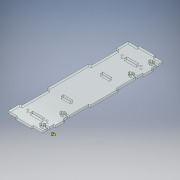
# Autodesk Inventor part: Cubierta_Ducto_Motor
Saved by Autodesk Inventor 2019 (Build 230136000, 136)
## iProperties
Created: 2020-04-03
Part Number: Cubierta_Ducto_Motor
Material: Generic
Document SubType Name: Modeling
Designer: Jurgen
Density: 1 g/cm^3
Appearance: Clear
Mass: 92.9987 g
Surface Area: 415.008 cm^2
Volume: 92.9987 cm^3
Author: Jurgen
Autodesk Inventor part; units mm, degrees
ref_plane "YZ Plane" through (0, 0, 0) normal (1, 0, 0) x (0, 1, 0)
ref_plane "XZ Plane" through (0, 0, 0) normal (0, 1, 0) x (-1, 0, 0)
ref_plane "XY Plane" through (0, 0, 0) normal (0, 0, 1) x (1, 0, 0)
sketch "Sketch1" plane through (0, 0, 0) normal (0, 1, 0) x (-1, 0, 0)
  line L0 (-25, -150) -> (25, -150)
  line L1 (25, 150) -> (-25, 150)
  line L2 (-25, 150) -> (-25, -150)
  line L3 (-25, -150) -> (25, 150) construction
  line L4 (25, -150) -> (-25, 150) construction
  line L5 (25, 150) -> (50, 150)
  line L6 (50, 150) -> (50, 105)
  line L7 (50, 105) -> (45, 105)
  line L8 (25, -150) -> (50, -150)
  line L9 (50, -150) -> (50, -105)
  line L10 (50, -105) -> (45, -105)
  line L11 (50, 105) -> (45, 105) construction
  line L12 (45, 105) -> (45, 45) construction
  line L13 (45, 45) -> (50, 45) construction
  line L14 (50, 45) -> (50, 105) construction
  line L15 (50, -105) -> (45, -105) construction
  line L16 (45, -105) -> (45, -45) construction
  line L17 (45, -45) -> (50, -45) construction
  line L18 (50, -45) -> (50, -105) construction
  line L19 (45, 45) -> (50, 45)
  line L20 (50, 45) -> (50, -45)
  line L21 (50, -45) -> (45, -45)
  line L22 (45, 105) -> (45, 45)
  line L23 (45, -45) -> (45, -105)
  point P0 (0, 0)
  dimension "d1" = 300
  dimension "d8" = 5
  dimension "d10" = 5
  dimension "d11" = 45
  dimension "d13" = 60
  dimension "d14" = 75
  dimension "d15" = 75
  dimension "d29" = 90
  dimension "d30" = 45
  dimension "d31" = 60
  constraints: 48 end point, 8 parallel, 6 horizontal, 5 perpendicular, 2 midpoint, 2 vertical
  measures "d1" distance of L1.start L0.end
  measures "d8" distance of L7.end L6.end
  measures "d10" distance of L10.end L9.end
  measures "d11" distance of L9.end L8.end
  measures "d13" distance of L16.end L15.end
  measures "d14" distance between parallel lines of L2 L9
  measures "d15" distance between parallel lines of L2 L6
  measures "d29" distance of L19.end L17.end
  measures "d30" distance of L5.end L6.end
  measures "d31" distance of L11.end L12.end
extrude "Extrusion1" add sketch "Sketch1" along normal blind 5
sketch "Sketch2" plane through (0, 5, 0) normal (0, 1, 0) x (1, 0, 0)
  line L0 (25, 150) -> (-50, 150) construction
  line L1 (-50, 150) -> (-50, 105) construction
  line L2 (-50, 105) -> (-45, 105) construction
  line L3 (-45, 105) -> (-45, 45) construction
  line L4 (-45, 45) -> (-50, 45) construction
  line L5 (-50, 45) -> (-50, -45) construction
  line L6 (-50, -45) -> (-45, -45) construction
  line L7 (-45, -45) -> (-45, -105) construction
  line L8 (-45, -105) -> (-50, -105) construction
  line L9 (-50, -105) -> (-50, -150) construction
  line L10 (-50, -150) -> (25, -150) construction
  line L11 (25, -150) -> (25, 150) construction
  line L12 (-50, -150) -> (25, -150)
  line L13 (25, -150) -> (25, -130)
  line L14 (25, -130) -> (-50, -130)
  line L15 (-50, -130) -> (-50, -150)
  line L16 (25, -150) -> (25, 150) projected
  line L17 (-50, 150) -> (25, 150)
  line L18 (25, 150) -> (25, 130)
  line L19 (25, 130) -> (-50, 130)
  line L20 (-50, 130) -> (-50, 150)
  point P0 (0, 0)
  dimension "d16" = 20
  dimension "d17" = 20
  constraints: 16 end point, 4 parallel, 2 horizontal, 2 perpendicular, 2 point on line
  measures "d16" distance of L13.end L12.end
  measures "d17" distance of L17.end L18.end
extrude "Extrusion2" cut sketch "Sketch2" against normal blind 5
sketch "Sketch3" plane through (0, 5, 0) normal (0, 1, 0) x (1, 0, 0)
  line L0 (-50, -130) -> (25, -130) construction
  line L1 (25, -130) -> (25, 130) construction
  line L2 (25, 130) -> (-50, 130) construction
  line L3 (-50, 130) -> (-50, 105) construction
  line L4 (-50, 105) -> (-45, 105) construction
  line L5 (-45, 105) -> (-45, 45) construction
  line L6 (-45, 45) -> (-50, 45) construction
  line L7 (-50, 45) -> (-50, -45) construction
  line L8 (-50, -45) -> (-45, -45) construction
  line L9 (-45, -45) -> (-45, -105) construction
  line L10 (-45, -105) -> (-50, -105) construction
  line L11 (-50, -105) -> (-50, -130) construction
  line L12 (2.5, 100) -> (-22.5, 100)
  line L13 (-22.5, 100) -> (-22.5, 95)
  line L14 (-22.5, 95) -> (2.5, 95)
  line L15 (2.5, 95) -> (2.5, 100)
  line L16 (2.5, -109) -> (-22.5, -109)
  line L17 (-22.5, -109) -> (-22.5, -104)
  line L18 (-22.5, -104) -> (2.5, -104)
  line L19 (2.5, -104) -> (2.5, -109)
  point P0 (0, 0)
  dimension "d20" = 25
  dimension "d21" = 5
  dimension "d22" = 22.5
  dimension "d23" = 35
  dimension "d26" = 5
  dimension "d27" = 25
  dimension "d28" = 26
  dimension "d32" = 22.5
  constraints: 16 end point, 2 parallel, 1 horizontal, 1 perpendicular
  measures "d20" distance of L14.end L13.end
  measures "d21" distance of L13.end L12.end
  measures "d22" distance between parallel lines of L1 L15
  measures "d23" distance between parallel lines of L2 L14
  measures "d26" distance of L18.end L19.end
  measures "d27" distance of L18.start L18.end
  measures "d28" distance between parallel lines of L0 L18
  measures "d32" distance between parallel lines of L1 L19
extrude "Extrusion3" cut sketch "Sketch3" against normal blind 5
sketch "Sketch4" plane through (0, 5, 0) normal (0, 1, 0) x (1, 0, 0)
  line L0 (-22.5, 95) -> (-22.5, 100) construction
  line L1 (-22.5, 100) -> (2.5, 100) construction
  line L2 (2.5, 100) -> (2.5, 95) construction
  line L3 (2.5, 95) -> (-22.5, 95) construction
  line L4 (2.5, -109) -> (-22.5, -109) construction
  line L5 (-22.5, -109) -> (-22.5, -104) construction
  line L6 (-22.5, -104) -> (2.5, -104) construction
  line L7 (2.5, -104) -> (2.5, -109) construction
  line L8 (-50, -130) -> (25, -130) construction
  line L9 (25, -130) -> (25, 130) construction
  line L10 (25, 130) -> (-50, 130) construction
  line L11 (-50, 130) -> (-50, 105) construction
  line L12 (-50, 105) -> (-45, 105) construction
  line L13 (-45, 105) -> (-45, 45) construction
  line L14 (-45, 45) -> (-50, 45) construction
  line L15 (-50, 45) -> (-50, -45) construction
  line L16 (-50, -45) -> (-45, -45) construction
  line L17 (-45, -45) -> (-45, -105) construction
  line L18 (-45, -105) -> (-50, -105) construction
  line L19 (-50, -105) -> (-50, -130) construction
  line L20 (2.5, 97.5) -> (25, 97.5) construction
  line L21 (-22.5, 97.5) -> (-45, 97.5) construction
  line L22 (-22.5, -104) -> (-22.5, -109) construction
  line L23 (-22.5, -106.5) -> (-50, -106.5) construction
  line L24 (2.5, -109) -> (2.5, -104) construction
  line L25 (2.5, -106.5) -> (25, -106.5) construction
  circle A0 centre (-30.5, -106.5) radius 2
  circle A1 centre (10.5, -106.5) radius 2
  circle A2 centre (-30.5, 97.5) radius 2
  circle A3 centre (10.5, 97.5) radius 2
  point P0 (0, 0)
  dimension "d33" = 4
  dimension "d34" = 4
  dimension "d35" = 4
  dimension "d36" = 4
  dimension "d37" = 8
  dimension "d38" = 8
  dimension "d39" = 8
  dimension "d40" = 8
  constraints: 10 point on line, 8 end point, 4 centre point, 4 midpoint, 1 horizontal, 1 perpendicular
  measures "d33" diameter of A0
  measures "d34" diameter of A1
  measures "d35" diameter of A2
  measures "d36" diameter of A3
  measures "d37" distance from line of L0 A2.centre
  measures "d38" distance from line of A3.centre L2
  measures "d39" distance from line of L5 A0.centre
  measures "d40" distance from line of A1.centre L24
extrude "Extrusion4" cut sketch "Sketch4" against normal blind 5
sketch "Sketch5" plane through (0, 5, 0) normal (0, 1, 0) x (1, 0, 0)
  circle A0 centre (-30.5, 97.5) radius 2 construction
  circle A1 centre (-30.5, -106.5) radius 2 construction
  circle A2 centre (10.5, -106.5) radius 2 construction
  circle A3 centre (10.5, 97.5) radius 2 construction
  line L0 (-22.5, 95) -> (-22.5, 100) construction
  line L1 (-22.5, 100) -> (2.5, 100) construction
  line L2 (2.5, 100) -> (2.5, 95) construction
  line L3 (2.5, 95) -> (-22.5, 95) construction
  line L4 (2.5, -109) -> (-22.5, -109) construction
  line L5 (-22.5, -109) -> (-22.5, -104) construction
  line L6 (-22.5, -104) -> (2.5, -104) construction
  line L7 (2.5, -104) -> (2.5, -109) construction
  line L8 (-50, -130) -> (25, -130) construction
  line L9 (25, -130) -> (25, 130) construction
  line L10 (25, 130) -> (-50, 130) construction
  line L11 (-50, 130) -> (-50, 105) construction
  line L12 (-50, 105) -> (-45, 105) construction
  line L13 (-45, 105) -> (-45, 45) construction
  line L14 (-45, 45) -> (-50, 45) construction
  line L15 (-50, 45) -> (-50, -45) construction
  line L16 (-50, -45) -> (-45, -45) construction
  line L17 (-45, -45) -> (-45, -105) construction
  line L18 (-45, -105) -> (-50, -105) construction
  line L19 (-50, -105) -> (-50, -130) construction
  line L20 (-45, 45) -> (25, 45) construction
  line L21 (-45, -45) -> (25, -45) construction
  line L22 (-20, -45) -> (0, -45)
  line L23 (0, -45) -> (0, -40)
  line L24 (0, -40) -> (-20, -40)
  line L25 (-20, -40) -> (-20, -45)
  line L26 (-50, 0) -> (25, 0) construction
  line L27 (-20, 45) -> (0, 45)
  line L28 (0, 45) -> (0, 40)
  line L29 (0, 40) -> (-20, 40)
  line L30 (-20, 40) -> (-20, 45)
  point P0 (0, 0)
  dimension "d43" = 20
  dimension "d44" = 5
  dimension "d45" = 25
  constraints: 22 end point, 4 symmetric about line, 3 point on line, 2 horizontal, 2 midpoint, 2 parallel, 2 perpendicular
  measures "d43" distance of L24.end L23.end
  measures "d44" distance of L23.end L22.end
  measures "d45" distance between parallel lines of L9 L23
extrude "Extrusion5" cut sketch "Sketch5" against normal blind 10
sketch "Sketch6" plane through (0, 5, 0) normal (0, 1, 0) x (1, 0, 0)
  line L0 (0, -40) -> (0, -45) construction
  line L1 (0, -45) -> (-20, -45) construction
  line L2 (-20, -45) -> (-20, -40) construction
  line L3 (-20, -40) -> (0, -40) construction
  line L4 (0, 45) -> (0, 40) construction
  line L5 (0, 40) -> (-20, 40) construction
  line L6 (-20, 40) -> (-20, 45) construction
  line L7 (-20, 45) -> (0, 45) construction
  circle A0 centre (-30.5, 97.5) radius 2 construction
  circle A1 centre (-30.5, -106.5) radius 2 construction
  circle A2 centre (10.5, -106.5) radius 2 construction
  circle A3 centre (10.5, 97.5) radius 2 construction
  line L8 (-22.5, 95) -> (-22.5, 100) construction
  line L9 (-22.5, 100) -> (2.5, 100) construction
  line L10 (2.5, 100) -> (2.5, 95) construction
  line L11 (2.5, 95) -> (-22.5, 95) construction
  line L12 (2.5, -109) -> (-22.5, -109) construction
  line L13 (-22.5, -109) -> (-22.5, -104) construction
  line L14 (-22.5, -104) -> (2.5, -104) construction
  line L15 (2.5, -104) -> (2.5, -109) construction
  line L16 (-50, -130) -> (25, -130) construction
  line L17 (25, -130) -> (25, 130) construction
  line L18 (25, 130) -> (-50, 130) construction
  line L19 (-50, 130) -> (-50, 105) construction
  line L20 (-50, 105) -> (-45, 105) construction
  line L21 (-45, 105) -> (-45, 45) construction
  line L22 (-45, 45) -> (-50, 45) construction
  line L23 (-50, 45) -> (-50, -45) construction
  line L24 (-50, -45) -> (-45, -45) construction
  line L25 (-45, -45) -> (-45, -105) construction
  line L26 (-45, -105) -> (-50, -105) construction
  line L27 (-50, -105) -> (-50, -130) construction
  line L28 (25, -130) -> (25, 130) construction
  line L29 (25, -120) -> (10, -120) construction
  line L30 (10, -120) -> (10, -116) construction
  line L31 (10, -116) -> (25, -116) construction
  line L32 (25, -116) -> (25, -120) construction
  line L33 (10, -118) -> (25, -118) construction
  line L34 (18, -114) -> (14, -114) construction
  line L35 (14, -114) -> (14, -122) construction
  line L36 (14, -122) -> (18, -122) construction
  line L37 (18, -122) -> (18, -114) construction
  line L38 (18, -114) -> (14, -122) construction
  line L39 (14, -114) -> (18, -122) construction
  line L40 (25, -116) -> (25, -120)
  line L41 (25, -120) -> (18, -120)
  line L42 (18, -120) -> (18, -122)
  line L43 (18, -122) -> (14, -122)
  line L44 (14, -122) -> (14, -120)
  line L45 (14, -120) -> (10, -120)
  line L46 (10, -120) -> (10, -116)
  line L47 (10, -116) -> (14, -116)
  line L48 (14, -116) -> (14, -114)
  line L49 (14, -114) -> (18, -114)
  line L50 (18, -114) -> (18, -116)
  line L51 (18, -116) -> (25, -116)
  line L52 (25, -76) -> (10, -76) construction
  line L53 (10, -76) -> (10, -72) construction
  line L54 (10, -72) -> (25, -72) construction
  line L55 (25, -72) -> (25, -76) construction
  line L56 (10, -74) -> (25, -74) construction
  line L57 (18, -70) -> (14, -70) construction
  line L58 (14, -70) -> (14, -78) construction
  line L59 (14, -78) -> (18, -78) construction
  line L60 (18, -78) -> (18, -70) construction
  line L61 (18, -70) -> (14, -78) construction
  line L62 (14, -70) -> (18, -78) construction
  line L63 (25, -72) -> (25, -76)
  line L64 (25, -76) -> (18, -76)
  line L65 (18, -76) -> (18, -78)
  line L66 (18, -78) -> (14, -78)
  line L67 (14, -78) -> (14, -76)
  line L68 (14, -76) -> (10, -76)
  line L69 (10, -76) -> (10, -72)
  line L70 (10, -72) -> (14, -72)
  line L71 (14, -72) -> (14, -70)
  line L72 (14, -70) -> (18, -70)
  line L73 (18, -70) -> (18, -72)
  line L74 (18, -72) -> (25, -72)
  line L75 (25, -106) -> (28.5, -106)
  line L76 (28.5, -106) -> (28.5, -86)
  line L77 (28.5, -86) -> (25, -86)
  line L78 (25, -86) -> (25, -106)
  line L79 (25, 72) -> (10, 72) construction
  line L80 (10, 72) -> (10, 76) construction
  line L81 (10, 76) -> (25, 76) construction
  line L82 (25, 76) -> (25, 72) construction
  line L83 (10, 74) -> (25, 74) construction
  line L84 (18, 78) -> (14, 78) construction
  line L85 (14, 78) -> (14, 70) construction
  line L86 (14, 70) -> (18, 70) construction
  line L87 (18, 70) -> (18, 78) construction
  line L88 (18, 78) -> (14, 70) construction
  line L89 (14, 78) -> (18, 70) construction
  line L90 (25, 76) -> (25, 72)
  line L91 (25, 72) -> (18, 72)
  line L92 (18, 72) -> (18, 70)
  line L93 (18, 70) -> (14, 70)
  line L94 (14, 70) -> (14, 72)
  line L95 (14, 72) -> (10, 72)
  line L96 (10, 72) -> (10, 76)
  line L97 (10, 76) -> (14, 76)
  line L98 (14, 76) -> (14, 78)
  line L99 (14, 78) -> (18, 78)
  line L100 (18, 78) -> (18, 76)
  line L101 (18, 76) -> (25, 76)
  line L102 (18, 122) -> (14, 122) construction
  line L103 (14, 122) -> (18, 122)
  line L104 (18, 122) -> (18, 120)
  line L105 (10, 120) -> (25, 120) construction
  line L106 (10, 118) -> (25, 118) construction
  line L107 (25, 116) -> (10, 116) construction
  line L108 (18, 114) -> (18, 122) construction
  line L109 (18, 122) -> (14, 114) construction
  line L110 (14, 122) -> (18, 114) construction
  line L111 (14, 122) -> (14, 114) construction
  line L112 (14, 114) -> (18, 114) construction
  line L113 (18, 114) -> (14, 114)
  line L114 (18, 116) -> (18, 114)
  line L115 (25, 116) -> (18, 116)
  line L116 (25, 120) -> (25, 116) construction
  line L117 (25, 120) -> (25, 116)
  line L118 (18, 120) -> (25, 120)
  line L119 (10, 116) -> (10, 120) construction
  line L120 (14, 114) -> (14, 116)
  line L121 (14, 120) -> (14, 122)
  line L122 (10, 120) -> (14, 120)
  line L123 (14, 116) -> (10, 116)
  line L124 (10, 116) -> (10, 120)
  line L125 (25, 86) -> (28.5, 86)
  line L126 (28.5, 86) -> (28.5, 106)
  line L127 (28.5, 106) -> (25, 106)
  line L128 (25, 106) -> (25, 86)
  line L129 (25, -30) -> (28.5, -30)
  line L130 (28.5, -30) -> (28.5, 30)
  line L131 (28.5, 30) -> (25, 30)
  line L132 (25, 30) -> (25, -30)
  line L133 (25, -130) -> (25, 130) projected
  point P0 (0, 0)
  point P1 (16, -118)
  point P2 (16, -74)
  point P3 (16, 74)
  point P4 (16, 118)
  dimension "d48" = 15
  dimension "d49" = 4
  dimension "d50" = 4
  dimension "d51" = 8
  dimension "d52" = 4
  dimension "d53" = 10
  dimension "d54" = 15
  dimension "d55" = 4
  dimension "d56" = 4
  dimension "d57" = 8
  dimension "d58" = 4
  dimension "d60" = 40
  dimension "d61" = 3.5
  dimension "d62" = 20
  dimension "d63" = 10
  dimension "d64" = 15
  dimension "d65" = 4
  dimension "d66" = 4
  dimension "d67" = 8
  dimension "d68" = 4
  dimension "d69" = 15
  dimension "d70" = 4
  dimension "d71" = 4
  dimension "d72" = 8
  dimension "d73" = 4
  dimension "d74" = 40
  dimension "d75" = 3.5
  dimension "d76" = 20
  dimension "d77" = 10
  dimension "d78" = 10
  dimension "d79" = 3.5
  dimension "d80" = 60
  dimension "d81" = 30
  constraints: 208 end point, 39 point on line, 23 perpendicular, 22 parallel, 16 midpoint, 11 horizontal, 9 collinear, 1 vertical, 1 other
  measures "d48" distance of L30.end L31.end
  measures "d49" distance of L29.end L30.end
  measures "d50" distance of L36.end L35.end
  measures "d51" distance of L35.end L34.end
  measures "d52" distance between parallel lines of L30 L35
  measures "d53" distance between parallel lines of L16 L29
  measures "d54" distance of L54.start L54.end
  measures "d55" distance of L52.end L54.start
  measures "d56" distance of L60.start L61.end
  measures "d57" distance of L61.end L57.end
  measures "d58" distance between parallel lines of L53 L58
  measures "d60" distance between parallel lines of L51 L64
  measures "d61" distance of L77.end L76.end
  measures "d62" distance of L76.end L75.end
  measures "d63" distance between parallel lines of L31 L75
  measures "d64" distance of L80.end L81.end
  measures "d65" distance of L80.start L80.end
  measures "d66" distance of L92.end L94.start
  measures "d67" distance of L94.start L98.end
  measures "d68" distance between parallel lines of L80 L85
  measures "d69" distance of L105.start L105.end
  measures "d70" distance of L107.end L105.start
  measures "d71" distance of L112.end L112.start
  measures "d72" distance of L112.start L102.end
  measures "d73" distance between parallel lines of L119 L111
  measures "d74" distance between parallel lines of L101 L115
  measures "d75" distance of L128.start L127.start
  measures "d76" distance of L127.start L126.start
  measures "d77" distance between parallel lines of L81 L125
  measures "d78" distance between parallel lines of L18 L118
  measures "d79" distance of L131.end L130.end
  measures "d80" distance of L130.end L129.end
  measures "d81" distance from line of point (0, 0) L129
extrude "Extrusion6" add sketch "Sketch6" against normal blind 5 contours L128 L127 L126 L125 | L132 L131 L130 L129 | L78 L77 L76 L75
sketch "Sketch8" plane through (0, 5, 0) normal (0, 1, 0) x (1, 0, 0)
  line L0 (0, -40) -> (0, -45) construction
  line L1 (0, -45) -> (-20, -45) construction
  line L2 (-20, -45) -> (-20, -40) construction
  line L3 (-20, -40) -> (0, -40) construction
  line L4 (0, 45) -> (0, 40) construction
  line L5 (0, 40) -> (-20, 40) construction
  line L6 (-20, 40) -> (-20, 45) construction
  line L7 (-20, 45) -> (0, 45) construction
  circle A0 centre (-30.5, 97.5) radius 2 construction
  circle A1 centre (-30.5, -106.5) radius 2 construction
  circle A2 centre (10.5, -106.5) radius 2 construction
  circle A3 centre (10.5, 97.5) radius 2 construction
  line L8 (-22.5, 95) -> (-22.5, 100) construction
  line L9 (-22.5, 100) -> (2.5, 100) construction
  line L10 (2.5, 100) -> (2.5, 95) construction
  line L11 (2.5, 95) -> (-22.5, 95) construction
  line L12 (2.5, -109) -> (-22.5, -109) construction
  line L13 (-22.5, -109) -> (-22.5, -104) construction
  line L14 (-22.5, -104) -> (2.5, -104) construction
  line L15 (2.5, -104) -> (2.5, -109) construction
  line L16 (-50, -130) -> (25, -130) construction
  line L17 (25, -130) -> (25, -106) construction
  line L18 (25, -106) -> (28.5, -106) construction
  line L19 (28.5, -106) -> (28.5, -86) construction
  line L20 (28.5, -86) -> (25, -86) construction
  line L21 (25, -86) -> (25, -30) construction
  line L22 (25, -30) -> (28.5, -30) construction
  line L23 (28.5, -30) -> (28.5, 30) construction
  line L24 (28.5, 30) -> (25, 30) construction
  line L25 (25, 30) -> (25, 86) construction
  line L26 (28.5, 86) -> (25, 86) construction
  line L27 (28.5, 106) -> (28.5, 86) construction
  line L28 (25, 106) -> (28.5, 106) construction
  line L29 (25, 106) -> (25, 130) construction
  line L30 (25, 130) -> (-50, 130) construction
  line L31 (-50, 130) -> (-50, 105) construction
  line L32 (-50, 105) -> (-45, 105) construction
  line L33 (-45, 105) -> (-45, 45) construction
  line L34 (-45, 45) -> (-50, 45) construction
  line L35 (-50, 45) -> (-50, -45) construction
  line L36 (-50, -45) -> (-45, -45) construction
  line L37 (-45, -45) -> (-45, -105) construction
  line L38 (-45, -105) -> (-50, -105) construction
  line L39 (-50, -105) -> (-50, -130) construction
  line L40 (25, -130) -> (25, -106) construction
  line L41 (25, -120) -> (8, -120) construction
  line L42 (8, -120) -> (8, -116) construction
  line L43 (8, -116) -> (25, -116) construction
  line L44 (25, -116) -> (25, -120) construction
  line L45 (8, -118) -> (25, -118) construction
  line L46 (16, -122) -> (12, -122) construction
  line L47 (12, -122) -> (12, -114) construction
  line L48 (12, -114) -> (16, -114) construction
  line L49 (16, -114) -> (16, -122) construction
  line L50 (16, -122) -> (12, -114) construction
  line L51 (12, -122) -> (16, -114) construction
  line L52 (25, -120) -> (16, -120)
  line L53 (16, -120) -> (16, -122)
  line L54 (16, -122) -> (12, -122)
  line L55 (12, -122) -> (12, -120)
  line L56 (12, -120) -> (8, -120)
  line L57 (8, -120) -> (8, -116)
  line L58 (8, -116) -> (12, -116)
  line L59 (12, -116) -> (12, -114)
  line L60 (12, -114) -> (16, -114)
  line L61 (16, -114) -> (16, -116)
  line L62 (16, -116) -> (25, -116)
  line L63 (25, -120) -> (25, -116)
  line L64 (25, -76) -> (8, -76) construction
  line L65 (8, -76) -> (8, -72) construction
  line L66 (8, -72) -> (25, -72) construction
  line L67 (25, -72) -> (25, -76) construction
  line L68 (8, -74) -> (25, -74) construction
  line L69 (16, -78) -> (12, -78) construction
  line L70 (12, -78) -> (12, -70) construction
  line L71 (12, -70) -> (16, -70) construction
  line L72 (16, -70) -> (16, -78) construction
  line L73 (16, -78) -> (12, -70) construction
  line L74 (12, -78) -> (16, -70) construction
  line L75 (25, -76) -> (16, -76)
  line L76 (16, -76) -> (16, -78)
  line L77 (16, -78) -> (12, -78)
  line L78 (12, -78) -> (12, -76)
  line L79 (12, -76) -> (8, -76)
  line L80 (8, -76) -> (8, -72)
  line L81 (8, -72) -> (12, -72)
  line L82 (12, -72) -> (12, -70)
  line L83 (12, -70) -> (16, -70)
  line L84 (16, -70) -> (16, -72)
  line L85 (16, -72) -> (25, -72)
  line L86 (25, -76) -> (25, -72)
  line L87 (25, 72) -> (8, 72) construction
  line L88 (8, 72) -> (8, 76) construction
  line L89 (8, 76) -> (25, 76) construction
  line L90 (25, 76) -> (25, 72) construction
  line L91 (8, 74) -> (25, 74) construction
  line L92 (16, 70) -> (12, 70) construction
  line L93 (12, 70) -> (12, 78) construction
  line L94 (12, 78) -> (16, 78) construction
  line L95 (16, 78) -> (16, 70) construction
  line L96 (16, 70) -> (12, 78) construction
  line L97 (12, 70) -> (16, 78) construction
  line L98 (25, 72) -> (16, 72)
  line L99 (16, 72) -> (16, 70)
  line L100 (16, 70) -> (12, 70)
  line L101 (12, 70) -> (12, 72)
  line L102 (12, 72) -> (8, 72)
  line L103 (8, 72) -> (8, 76)
  line L104 (8, 76) -> (12, 76)
  line L105 (12, 76) -> (12, 78)
  line L106 (12, 78) -> (16, 78)
  line L107 (16, 78) -> (16, 76)
  line L108 (16, 76) -> (25, 76)
  line L109 (25, 72) -> (25, 76)
  line L110 (25, 116) -> (8, 116) construction
  line L111 (8, 116) -> (8, 120) construction
  line L112 (8, 120) -> (25, 120) construction
  line L113 (25, 120) -> (25, 116) construction
  line L114 (8, 118) -> (25, 118) construction
  line L115 (16, 114) -> (12, 114) construction
  line L116 (12, 114) -> (12, 122) construction
  line L117 (12, 122) -> (16, 122) construction
  line L118 (16, 122) -> (16, 114) construction
  line L119 (16, 114) -> (12, 122) construction
  line L120 (12, 114) -> (16, 122) construction
  line L121 (25, 116) -> (16, 116)
  line L122 (16, 116) -> (16, 114)
  line L123 (16, 114) -> (12, 114)
  line L124 (12, 114) -> (12, 116)
  line L125 (12, 116) -> (8, 116)
  line L126 (8, 116) -> (8, 120)
  line L127 (8, 120) -> (12, 120)
  line L128 (12, 120) -> (12, 122)
  line L129 (12, 122) -> (16, 122)
  line L130 (16, 122) -> (16, 120)
  line L131 (16, 120) -> (25, 120)
  line L132 (25, 116) -> (25, 120)
  point P0 (14, -118)
  point P1 (14, -74)
  point P2 (14, 74)
  point P3 (14, 118)
  dimension "d152" = 17
  dimension "d153" = 4
  dimension "d154" = 4
  dimension "d155" = 8
  dimension "d156" = 10
  dimension "d157" = 17
  dimension "d158" = 4
  dimension "d159" = 4
  dimension "d160" = 8
  dimension "d161" = 17
  dimension "d162" = 4
  dimension "d163" = 4
  dimension "d164" = 8
  dimension "d165" = 17
  dimension "d166" = 4
  dimension "d167" = 4
  dimension "d168" = 8
  dimension "d169" = 10
  dimension "d170" = 10
  dimension "d171" = 10
  dimension "d182" = 4
  dimension "d183" = 0
  dimension "d184" = 4
  dimension "d185" = 0
  dimension "d186" = 4
  dimension "d187" = 0
  dimension "d188" = 4
  constraints: 184 end point, 41 point on line, 28 perpendicular, 16 midpoint, 16 parallel, 8 collinear, 8 horizontal
  measures "d152" distance of L42.end L43.end
  measures "d153" distance of L41.end L42.end
  measures "d154" distance of L47.end L48.end
  measures "d155" distance of L46.end L47.end
  measures "d156" distance between parallel lines of L16 L41
  measures "d157" distance of L81.start L66.end
  measures "d158" distance of L79.end L81.start
  measures "d159" distance of L71.start L84.start
  measures "d160" distance of L77.end L71.start
  measures "d161" distance of L104.start L89.end
  measures "d162" distance of L102.end L104.start
  measures "d163" distance of L94.start L107.start
  measures "d164" distance of L100.end L94.start
  measures "d165" distance of L127.start L112.end
  measures "d166" distance of L125.end L127.start
  measures "d167" distance of L117.start L130.start
  measures "d168" distance of L123.end L117.start
  measures "d169" distance between parallel lines of L64 L20
  measures "d170" distance between parallel lines of L26 L89
  measures "d171" distance between parallel lines of L28 L110
  measures "d182" distance between parallel lines of L42 L59
  measures "d183" distance from line of L21 L68.end
  measures "d184" distance between parallel lines of L65 L70
  measures "d185" distance from line of L25 L91.end
  measures "d186" distance between parallel lines of L88 L105
  measures "d187" distance between parallel lines of L29 L132
  measures "d188" distance between parallel lines of L126 L124
extrude "Extrusion7" cut sketch "Sketch8" against normal blind 10
sketch "Sketch9" plane through (0, 5, 0) normal (0, 1, 0) x (1, 0, 0)
  line L0 (16, 76) -> (25, 76) construction
  line L1 (25, 76) -> (25, 86) construction
  line L2 (28.5, 86) -> (25, 86) construction
  line L3 (28.5, 106) -> (28.5, 86) construction
  line L4 (25, 106) -> (28.5, 106) construction
  line L5 (25, 106) -> (25, 116) construction
  line L6 (25, 116) -> (16, 116) construction
  line L7 (16, 116) -> (16, 114) construction
  line L8 (16, 114) -> (12, 114) construction
  line L9 (12, 114) -> (12, 116) construction
  line L10 (12, 116) -> (8, 116) construction
  line L11 (8, 116) -> (8, 120) construction
  line L12 (8, 120) -> (12, 120) construction
  line L13 (12, 120) -> (12, 122) construction
  line L14 (12, 122) -> (16, 122) construction
  line L15 (16, 122) -> (16, 120) construction
  line L16 (16, 120) -> (25, 120) construction
  line L17 (25, 120) -> (25, 130) construction
  line L18 (25, 130) -> (-50, 130) construction
  line L19 (-50, 130) -> (-50, 105) construction
  line L20 (-50, 105) -> (-45, 105) construction
  line L21 (-45, 105) -> (-45, 45) construction
  line L22 (-45, 45) -> (-50, 45) construction
  line L23 (-50, 45) -> (-50, -45) construction
  line L24 (-50, -45) -> (-45, -45) construction
  line L25 (-45, -45) -> (-45, -105) construction
  line L26 (-45, -105) -> (-50, -105) construction
  line L27 (-50, -105) -> (-50, -130) construction
  line L28 (-50, -130) -> (25, -130) construction
  line L29 (25, -130) -> (25, -120) construction
  line L30 (25, -120) -> (16, -120) construction
  line L31 (16, -120) -> (16, -122) construction
  line L32 (16, -122) -> (12, -122) construction
  line L33 (12, -122) -> (12, -120) construction
  line L34 (12, -120) -> (8, -120) construction
  line L35 (8, -120) -> (8, -116) construction
  line L36 (8, -116) -> (12, -116) construction
  line L37 (12, -116) -> (12, -114) construction
  line L38 (12, -114) -> (16, -114) construction
  line L39 (16, -114) -> (16, -116) construction
  line L40 (16, -116) -> (25, -116) construction
  line L41 (25, -116) -> (25, -106) construction
  line L42 (25, -106) -> (28.5, -106) construction
  line L43 (28.5, -106) -> (28.5, -86) construction
  line L44 (28.5, -86) -> (25, -86) construction
  line L45 (25, -86) -> (25, -76) construction
  line L46 (25, -76) -> (16, -76) construction
  line L47 (16, -76) -> (16, -78) construction
  line L48 (16, -78) -> (12, -78) construction
  line L49 (12, -78) -> (12, -76) construction
  line L50 (12, -76) -> (8, -76) construction
  line L51 (8, -76) -> (8, -72) construction
  line L52 (8, -72) -> (12, -72) construction
  line L53 (12, -72) -> (12, -70) construction
  line L54 (12, -70) -> (16, -70) construction
  line L55 (16, -70) -> (16, -72) construction
  line L56 (16, -72) -> (25, -72) construction
  line L57 (25, -72) -> (25, -30) construction
  line L58 (25, -30) -> (28.5, -30) construction
  line L59 (28.5, -30) -> (28.5, 30) construction
  line L60 (28.5, 30) -> (25, 30) construction
  line L61 (25, 30) -> (25, 72) construction
  line L62 (25, 72) -> (16, 72) construction
  line L63 (16, 72) -> (16, 70) construction
  line L64 (16, 70) -> (12, 70) construction
  line L65 (12, 70) -> (12, 72) construction
  line L66 (12, 72) -> (8, 72) construction
  line L67 (8, 72) -> (8, 76) construction
  line L68 (8, 76) -> (12, 76) construction
  line L69 (12, 76) -> (12, 78) construction
  line L70 (12, 78) -> (16, 78) construction
  line L71 (16, 78) -> (16, 76) construction
  line L72 (0, -40) -> (0, -45) construction
  line L73 (0, -45) -> (-20, -45) construction
  line L74 (-20, -45) -> (-20, -40) construction
  line L75 (-20, -40) -> (0, -40) construction
  line L76 (0, 45) -> (0, 40) construction
  line L77 (0, 40) -> (-20, 40) construction
  line L78 (-20, 40) -> (-20, 45) construction
  line L79 (-20, 45) -> (0, 45) construction
  circle A0 centre (-30.5, 97.5) radius 2 construction
  circle A1 centre (-30.5, -106.5) radius 2 construction
  circle A2 centre (10.5, -106.5) radius 2 construction
  circle A3 centre (10.5, 97.5) radius 2 construction
  line L80 (-22.5, 95) -> (-22.5, 100) construction
  line L81 (-22.5, 100) -> (2.5, 100) construction
  line L82 (2.5, 100) -> (2.5, 95) construction
  line L83 (2.5, 95) -> (-22.5, 95) construction
  line L84 (2.5, -109) -> (-22.5, -109) construction
  line L85 (-22.5, -109) -> (-22.5, -104) construction
  line L86 (-22.5, -104) -> (2.5, -104) construction
  line L87 (2.5, -104) -> (2.5, -109) construction
  line L88 (-30, -130) -> (5, -130)
  line L89 (5, -130) -> (5, -133.5)
  line L90 (5, -133.5) -> (-30, -133.5)
  line L91 (-30, -133.5) -> (-30, -130)
  line L92 (-30, 130) -> (5, 130)
  line L93 (5, 130) -> (5, 133.5)
  line L94 (5, 133.5) -> (-30, 133.5)
  line L95 (-30, 133.5) -> (-30, 130)
  point P0 (0, 0)
  dimension "d174" = 35
  dimension "d175" = 3.5
  dimension "d176" = 35
  dimension "d177" = 3.5
  dimension "d178" = 20
  dimension "d179" = 20
  constraints: 16 end point, 4 parallel, 2 horizontal, 2 perpendicular, 2 point on line
  measures "d174" distance of L89.end L90.end
  measures "d175" distance of L88.end L89.end
  measures "d176" distance of L94.end L93.end
  measures "d177" distance of L93.end L92.end
  measures "d178" distance between parallel lines of L27 L91
  measures "d179" distance between parallel lines of L95 L19
extrude "Extrusion8" add sketch "Sketch9" against normal blind 5
body "Solid1"
